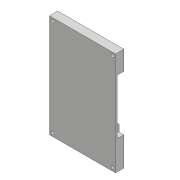
# Autodesk Inventor part: DE10-Nano
Saved by Autodesk Inventor 2018 (Build 220112000, 112)
## iProperties
Created: 2019-08-31
Part Number: DE10-Nano
Material: Generic
Document SubType Name: Modeling
Designer: Clevo
Density: 1 g/cm^3
Appearance: Default
Author: Clevo
Autodesk Inventor part; units mm, degrees
ref_plane "YZ Plane" through (0, 0, 0) normal (1, 0, 0) x (0, 1, 0)
ref_plane "XZ Plane" through (0, 0, 0) normal (0, 1, 0) x (-1, 0, 0)
ref_plane "XY Plane" through (0, 0, 0) normal (0, 0, 1) x (1, 0, 0)
sketch "Sketch1" plane through (0, 0, 0) normal (0, 1, 0) x (-1, 0, 0)
  line L0 (-34.295, -53.46) -> (34.295, -53.46)
  line L1 (34.295, -53.46) -> (34.295, 53.46)
  line L2 (34.295, 53.46) -> (-34.295, 53.46)
  line L3 (-34.295, 53.46) -> (-34.295, -53.46)
  line L4 (-34.295, -53.46) -> (34.295, 53.46) construction
  line L5 (34.295, -53.46) -> (-34.295, 53.46) construction
  point P0 (0, 0)
  dimension "d0" = 106.92
  dimension "d1" = 68.59
  constraints: 12 end point, 2 midpoint, 2 parallel, 1 horizontal, 1 perpendicular
  measures "d0" distance of L0.end L1.end
  measures "d1" distance of L1.end L2.end
extrude "Extrusion1" add sketch "Sketch1" along normal blind 1.6
sketch "Sketch2" plane through (0, 1.6, 0) normal (0, 1, 0) x (1, 0, 0)
  line L0 (-34.295, 53.46) -> (-34.295, -53.46) projected
  line L1 (34.295, -53.46) -> (34.295, 53.46) projected
  line L2 (-34.295, -53.46) -> (34.295, -53.46)
  line L3 (34.295, -53.46) -> (34.295, -33.46)
  line L4 (34.295, -33.46) -> (-34.295, -33.46)
  line L5 (-34.295, -33.46) -> (-34.295, -53.46)
  line L6 (34.295, 53.46) -> (-34.295, 53.46) projected
  line L7 (34.295, 53.46) -> (-34.295, 53.46)
  line L8 (-34.295, 53.46) -> (-34.295, 23.46)
  line L9 (-34.295, 23.46) -> (34.295, 23.46)
  line L10 (34.295, 23.46) -> (34.295, 53.46)
  point P0 (0, 0)
  dimension "d4" = 20
  dimension "d5" = 30
  constraints: 16 end point, 4 parallel, 2 horizontal, 2 perpendicular, 2 point on line
  measures "d4" distance between parallel lines of L2 L4
  measures "d5" distance between parallel lines of L6 L9
extrude "Extrusion2" add sketch "Sketch2" along normal blind 7 contours L6 L1 L9 L0 | L4 L1 L2 L0
sketch "Sketch3" plane through (0, 8.6, 0) normal (0, 1, 0) x (1, 0, 0)
  line L0 (34.295, 23.46) -> (-34.295, 23.46) projected
  line L1 (22.365, 53.46) -> (6.365, 53.46)
  line L2 (6.365, 53.46) -> (6.365, 23.46)
  line L3 (6.365, 23.46) -> (22.365, 23.46)
  line L4 (22.365, 23.46) -> (22.365, 53.46)
  line L5 (22.365, 53.46) -> (6.365, 23.46) construction
  line L6 (6.365, 53.46) -> (22.365, 23.46) construction
  line L7 (34.295, 53.46) -> (-34.295, 53.46) projected
  line L8 (34.295, 23.46) -> (34.295, 53.46) projected
  point P0 (0, 0)
  point P1 (14.365, 38.46)
  dimension "d8" = 19.93
  dimension "d9" = 16
  constraints: 12 end point, 2 midpoint, 2 parallel, 1 collinear, 1 horizontal, 1 perpendicular, 1 point on line
  measures "d8" distance from line of L8 point (14.365, 38.46)
  measures "d9" distance of L1.start L1.end
extrude "Extrusion3" add sketch "Sketch3" along normal blind 7 contours L0 L2 L1 L4
sketch "Sketch4" plane through (34.295, 0, -53.46) normal (0, 0, -1) x (-1, 0, 0)
  line L0 (13.93, 13.6) -> (25.93, 13.6)
  line L1 (25.93, 13.6) -> (25.93, 3.6)
  line L2 (25.93, 3.6) -> (13.93, 3.6)
  line L3 (13.93, 3.6) -> (13.93, 13.6)
  line L4 (11.93, 15.6) -> (27.93, 15.6) projected
  point P0 (34.295, 0)
  point P1 (25.93, 8.6)
  point P2 (27.93, 8.6)
  point P3 (19.93, 13.6)
  point P4 (19.93, 15.6)
  dimension "d12" = 12
  dimension "d13" = 10
  constraints: 8 end point, 3 midpoint, 2 parallel, 1 horizontal, 1 horizontal alignment, 1 perpendicular, 1 vertical alignment
  measures "d12" distance of L0.start L0.end
  measures "d13" distance of L0.end L1.end
extrude "Extrusion4" cut sketch "Sketch4" against normal blind 7
sketch "Sketch5" plane through (0, 8.6, 0) normal (0, 1, 0) x (1, 0, 0)
  line L0 (-31.115, -50.28) -> (31.115, -50.28)
  line L1 (31.115, -50.28) -> (31.115, 50.16)
  line L2 (31.115, 50.16) -> (-31.115, 50.16)
  line L3 (-31.115, 50.16) -> (-31.115, -50.28)
  line L4 (-34.295, -53.46) -> (34.295, -53.46) projected
  line L5 (34.295, -53.46) -> (34.295, -33.46) projected
  line L6 (-34.295, -33.46) -> (-34.295, -53.46) projected
  line L7 (6.365, 53.46) -> (-34.295, 53.46) projected
  point P0 (0, 0)
  dimension "d16" = 3.18
  dimension "d17" = 3.18
  dimension "d18" = 3.18
  dimension "d19" = 3.3
  constraints: 8 end point, 2 parallel, 1 horizontal, 1 perpendicular
  measures "d16" distance between parallel lines of L4 L0
  measures "d17" distance between parallel lines of L5 L1
  measures "d18" distance between parallel lines of L6 L3
  measures "d19" distance between parallel lines of L7 L2
hole "Hole1" at (-31.115, 8.6, 50.28) at (-31.115, 8.6, -50.16) at (31.115, 8.6, -50.16) at (31.115, 8.6, 50.28) direction (0, -1, 0) diameter 3.2 end through all clearance for "Flat Head Machine Screw" size "M3" standard "Ansi Metric M Profile"
sketch "Sketch6" plane through (0, 1.6, 0) normal (0, 1, 0) x (1, 0, 0)
  line L0 (-18, -12) -> (6, -12)
  line L1 (6, -12) -> (6, 12)
  line L2 (6, 12) -> (-18, 12)
  line L3 (-18, 12) -> (-18, -12)
  line L4 (-18, -12) -> (6, 12) construction
  line L5 (6, -12) -> (-18, 12) construction
  point P0 (0, 0)
  point P1 (-6, 0)
  point P2 (-6, 0)
  dimension "d27" = 24
  dimension "d28" = 24
  dimension "d29" = 6
  constraints: 12 end point, 3 midpoint, 2 parallel, 1 horizontal, 1 horizontal alignment, 1 perpendicular
  measures "d27" distance of L1.end L2.end
  measures "d28" distance of L2.end L0.start
  measures "d29" distance of point (0, 0) point (-6, 0)
extrude "Extrusion5" add sketch "Sketch6" along normal blind 3
equation "\"d28\" = d27"
body "Solid1"
